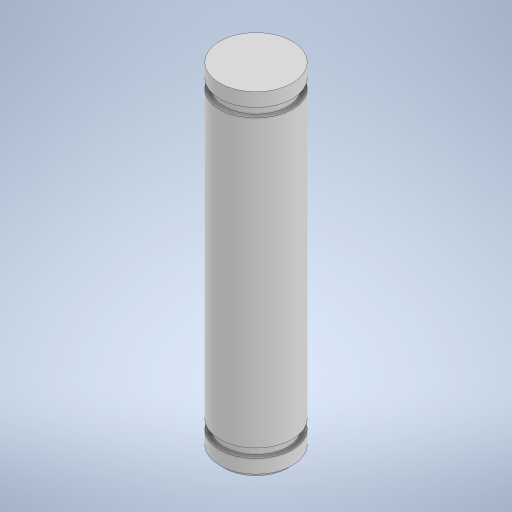
# Autodesk Inventor part: Part1
Saved by Autodesk Inventor 2023 (Build 270158000, 158)
## iProperties
Created: 2023-10-05
Part Number: Part1
Material: Generic
Document SubType Name: Modeling
Designer: huy20
Density: 1 g/cm^3
Appearance: Default
Author: huy20
Autodesk Inventor part; units mm, degrees
ref_plane "YZ Plane" through (0, 0, 0) normal (1, 0, 0) x (0, 1, 0)
ref_plane "XZ Plane" through (0, 0, 0) normal (0, 1, 0) x (-1, 0, 0)
ref_plane "XY Plane" through (0, 0, 0) normal (0, 0, 1) x (1, 0, 0)
sketch "Sketch1" plane through (0, 0, 0) normal (0, 1, 0) x (-1, 0, 0)
  circle A0 centre (0, 0) radius 4
  dimension "d0" = 8
  constraints: 1 centre point, 1 coincident
  measures "d0" diameter of A0
extrude "Extrusion1" add sketch "Sketch1" along normal blind 37
chamfer "Chamfer1" distance 0.5 angle 45 1 edges at (4, 0, 0)
sketch "Sketch2" plane through (0, 0, 0) normal (0, 0, 1) x (1, 0, 0)
  line L0 (-4, 0.5) -> (-4, 37) construction
  line L1 (-3.5, 0) -> (-4, 0.5) construction
  line L2 (-4, 0.5) -> (4, 0.5) construction
  line L3 (3.5, 0) -> (-3.5, 0) construction
  line L4 (4, 37) -> (-4, 37) projected
  line L5 (-4, 0.5) -> (4, 0.5) construction
  line L6 (3.5, 0) -> (4, 0.5) construction
  line L7 (4, 0.5) -> (4, 37) construction
  line L8 (4, 3) -> (3.5, 3)
  line L9 (3.5, 3) -> (3.5, 2)
  line L10 (3.5, 2) -> (4, 2)
  line L11 (4, 2) -> (4, 3)
  line L12 (0, -7.4) -> (0, 44.4) projected
  point P0 (0, 0)
  dimension "d6" = 2
  dimension "d7" = 1
  dimension "d8" = 0.5
  constraints: 8 end point, 2 parallel, 1 horizontal, 1 perpendicular, 1 point on line
  measures "d6" distance between parallel lines of L10 L3
  measures "d7" distance between parallel lines of L8 L10
  measures "d8" distance between parallel lines of L7 L9
revolve "Revolution1" cut sketch "Sketch2" angle 360 about axis through (0, -10, 0) along (0, 1, 0)
sketch "Sketch3" plane through (0, 0, 0) normal (1, 0, 0) x (0, 1, 0)
  line L0 (37, -4) -> (37, 4) construction
  line L1 (3, -4) -> (3, 4) construction
  line L2 (37, -4) -> (37, 4) construction
  line L3 (3, -4) -> (3, 4) construction
  line L4 (37, -4) -> (37, 4) construction
  line L5 (3, 4) -> (37, 4) construction
  line L6 (35.5, 4) -> (34.5, 4)
  line L7 (34.5, 4) -> (34.5, 3.5)
  line L8 (34.5, 3.5) -> (35.5, 3.5)
  line L9 (35.5, 3.5) -> (35.5, 4)
  line L10 (-7.4, 0) -> (44.4, 0) projected
  point P0 (0, 0)
  dimension "d10" = 1.5
  dimension "d11" = 1
  dimension "d12" = 0.5
  constraints: 8 end point, 2 parallel, 1 horizontal, 1 perpendicular, 1 point on line
  measures "d10" distance between parallel lines of L9 L0
  measures "d11" distance between parallel lines of L7 L9
  measures "d12" distance between parallel lines of L5 L8
revolve "Revolution2" cut sketch "Sketch3" angle 360 about axis through (0, -10, 0) along (0, 1, 0)
body "Solid1"
